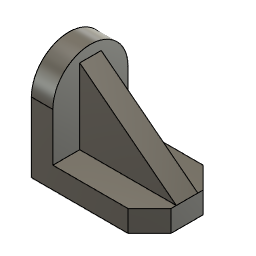
A1 (Autodesk Fusion 360 design; units mm, degrees)
Autodesk Fusion 360 part; units mm, degrees
sketch "Bottom part" plane through (0, 0, 0) normal (0, 1, 0) x (1, 0, 0)
  line L0 (-33, 21) -> (33, 21)
  line L1 (33, 21) -> (33, -21)
  line L2 (33, -21) -> (-33, -21)
  line L3 (-33, -21) -> (-33, 21)
  line L4 (-33, 21) -> (33, -21) construction
  line L5 (33, 21) -> (-33, -21) construction
  dimension "d1" = 66
  dimension "d2" = 42
  constraint horizontal L0
  constraint perpendicular L0 L1
  constraint parallel L0 L2
  constraint parallel L1 L3
  constraint coincident L4 origin
  constraint coincident L5 origin
  measures "d1" distance of L1.end L2.end
  measures "d2" distance of L0.end L1.end
extrude "Extrude1" add sketch "Bottom part" along normal blind 12 makes body 1
chamfer "Chamfer1" distance 12 angle 45 2 edges at (33, 6, 21) (33, 6, -21) on bodies 1
sketch "Vertical Part" plane through (0, 12, 0) normal (0, 1, 0) x (-1, 0, 0)
  line L0 (-33, -9) -> (-21, -21)
  line L1 (-21, -21) -> (33, -21)
  line L2 (33, -21) -> (33, 21)
  line L3 (33, 21) -> (-21, 21)
  line L4 (-21, 21) -> (-33, 9)
  line L5 (-33, 9) -> (-33, -9)
  line L6 (33, 21) -> (21, 21)
  line L7 (21, 21) -> (21, -21)
  line L8 (21, -21) -> (33, -21)
  line L9 (33, -21) -> (33, 21)
  dimension "d6" = 12
  dimension "d7" = 42
  constraint horizontal L6
  constraint vertical L7
  constraint horizontal L8
  constraint vertical L9
  constraint coincident L2.end L3.start
  measures "d6" distance of L2.end L6.end
  measures "d7" distance of L2.end L1.end
extrude "Extrude2" add sketch "Vertical Part" along normal blind 48 contours L1 L2 L3 L6 L7 L8 L9 bodies 1
fillet "Fillet1" radius 21 2 edges at (-27, 60, 21) (-27, 60, -21) on bodies 1
sketch "Triangular Part" plane through (0, 0, 0) normal (0, 0, 1) x (1, 0, 0)
  line L0 (-20.9988, 12.0018) -> (33.0012, 12.0018)
  line L1 (33.0012, 12.0018) -> (-20.9988, 54.0018)
  line L2 (-20.9988, 54.0018) -> (-20.9988, 12.0018)
  dimension "d11" = 42
  dimension "d12" = 54
  constraint horizontal L0
  constraint perpendicular L0 L2
  measures "d11" distance of L0.start L1.end
  measures "d12" distance of L0.start L0.end
extrude "Extrude3" add sketch "Triangular Part" along normal mid plane 12 separate body makes body 2
combine "Combine1" operation add target body 2 tool bodies 1 makes body 3 at (-15, 0, -7)
combine "Combine2" operation add target body 3 tool bodies 2 makes body 4 at (-2.9988, 26.0018, 6)
move_face "MoveFace1" by (0.0095, -0.0064, 0) 1 faces at (-2.9988, 26.0018, 6) on bodies 4
move_body "Move1" bodies 4 to x (1, 0, 0) y (0, 1, 0) z (0, 0, 1) at (-0.0013, -0.0019, 0)
combine "Combine3" operation add target body 3 tool bodies 4
equation "d8 = 60 mm - 12 mm"
named bodies: "A1"
